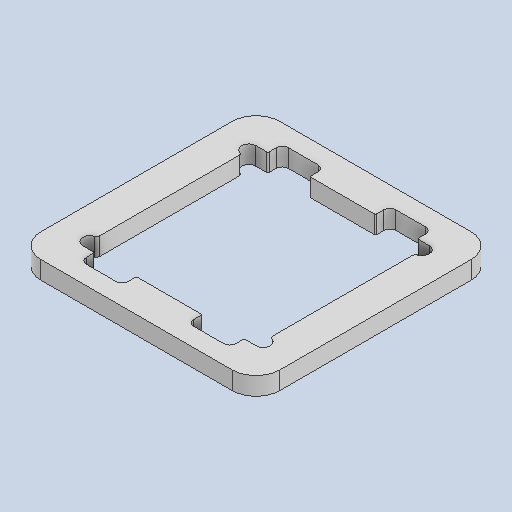
# Autodesk Inventor part: test switch hole
Saved by Autodesk Inventor 2025.2 (Build 292293000, 293)
## iProperties
Created: 2024-03-08
Part Number: test switch hole
Material: Generic
Document SubType Name: Modeling
Designer: mirun
Density: 1 g/cm^3
Appearance: Default
Author: mirun
Autodesk Inventor part; units mm, degrees
ref_plane "YZ Plane" through (0, 0, 0) normal (1, 0, 0) x (0, 1, 0)
ref_plane "XZ Plane" through (0, 0, 0) normal (0, 1, 0) x (-1, 0, 0)
ref_plane "XY Plane" through (0, 0, 0) normal (0, 0, 1) x (1, 0, 0)
sketch "Sketch1" plane through (0, 0, 0) normal (0, 1, 0) x (-1, 0, 0)
  line L0 (7.25, 5.8376) -> (7.25, -5.8376)
  line L1 (-7.25, -5.8376) -> (-7.25, 5.8376)
  line L2 (-7.25, 7.25) -> (7.25, -7.25) construction
  line L3 (7.25, 7.25) -> (-7.25, -7.25) construction
  line L4 (6.25, 7.25) -> (2.75, 7.25) construction
  line L5 (2.75, 7.35) -> (2.75, 7.95)
  line L6 (3.25, 8.45) -> (5.75, 8.45)
  line L7 (6.25, 7.95) -> (6.25, 7.35)
  arc A0 (7.4265, 6.0765) -> (7.25, 7.25) centre (7.25, 6.65) ccw
  line L8 (-7.25, 7.25) -> (2.65, 7.25)
  line L9 (6.35, 7.25) -> (7.25, 7.25)
  arc A1 (6.25, 7.35) -> (6.35, 7.25) centre (6.35, 7.35) ccw
  arc A2 (2.65, 7.25) -> (2.75, 7.35) centre (2.65, 7.35) ccw
  arc A3 (6.25, 7.95) -> (5.75, 8.45) centre (5.75, 7.95) ccw
  arc A4 (3.25, 8.45) -> (2.75, 7.95) centre (3.25, 7.95) ccw
  arc A5 (7.4265, 6.0765) -> (7.25, 5.8376) centre (7.5, 5.8376) ccw
  line L10 (0, 0) -> (2.8942, 0)
  line L11 (0, 0) -> (0, -4.9214)
  line L12 (7.25, -7.25) -> (-7.25, 7.25) construction
  line L13 (6.25, -7.25) -> (2.75, -7.25) construction
  line L14 (2.75, -7.35) -> (2.75, -7.95)
  line L15 (3.25, -8.45) -> (5.75, -8.45)
  line L16 (6.25, -7.95) -> (6.25, -7.35)
  arc A6 (7.25, -7.25) -> (7.4265, -6.0765) centre (7.25, -6.65) ccw
  line L17 (6.35, -7.25) -> (7.25, -7.25)
  arc A7 (6.35, -7.25) -> (6.25, -7.35) centre (6.35, -7.35) ccw
  arc A8 (2.75, -7.35) -> (2.65, -7.25) centre (2.65, -7.35) ccw
  arc A9 (5.75, -8.45) -> (6.25, -7.95) centre (5.75, -7.95) ccw
  arc A10 (2.75, -7.95) -> (3.25, -8.45) centre (3.25, -7.95) ccw
  arc A11 (7.25, -5.8376) -> (7.4265, -6.0765) centre (7.5, -5.8376) ccw
  line L18 (7.25, -7.25) -> (6.35, -7.25)
  line L19 (-6.25, 7.25) -> (-2.75, 7.25) construction
  line L20 (-2.75, 7.35) -> (-2.75, 7.95)
  line L21 (-3.25, 8.45) -> (-5.75, 8.45)
  line L22 (-6.25, 7.95) -> (-6.25, 7.35)
  arc A12 (-7.25, 7.25) -> (-7.4265, 6.0765) centre (-7.25, 6.65) ccw
  line L23 (-6.35, 7.25) -> (-7.25, 7.25)
  arc A13 (-6.35, 7.25) -> (-6.25, 7.35) centre (-6.35, 7.35) ccw
  arc A14 (-2.75, 7.35) -> (-2.65, 7.25) centre (-2.65, 7.35) ccw
  arc A15 (-5.75, 8.45) -> (-6.25, 7.95) centre (-5.75, 7.95) ccw
  arc A16 (-2.75, 7.95) -> (-3.25, 8.45) centre (-3.25, 7.95) ccw
  arc A17 (-7.25, 5.8376) -> (-7.4265, 6.0765) centre (-7.5, 5.8376) ccw
  arc A18 (-7.4265, -6.0765) -> (-7.25, -5.8376) centre (-7.5, -5.8376) ccw
  arc A19 (-7.4265, -6.0765) -> (-7.25, -7.25) centre (-7.25, -6.65) ccw
  line L24 (-6.35, -7.25) -> (-7.25, -7.25)
  line L25 (-7.25, -7.25) -> (7.25, 7.25) construction
  arc A20 (-6.25, -7.35) -> (-6.35, -7.25) centre (-6.35, -7.35) ccw
  line L26 (-6.25, -7.95) -> (-6.25, -7.35)
  arc A21 (-6.25, -7.95) -> (-5.75, -8.45) centre (-5.75, -7.95) ccw
  line L27 (-6.25, -7.25) -> (-2.75, -7.25) construction
  line L28 (-3.25, -8.45) -> (-5.75, -8.45)
  arc A22 (-2.65, -7.25) -> (-2.75, -7.35) centre (-2.65, -7.35) ccw
  line L29 (-2.75, -7.35) -> (-2.75, -7.95)
  arc A23 (-3.25, -8.45) -> (-2.75, -7.95) centre (-3.25, -7.95) ccw
  line L30 (-7.25, -7.25) -> (-6.35, -7.25)
  line L31 (2.65, -7.25) -> (-2.65, -7.25)
  line L32 (-6.35, -7.25) -> (-7.25, -7.25)
  line L33 (8, -10) -> (-8, -10)
  line L34 (-10, -8) -> (-10, 8)
  line L35 (-8, 10) -> (8, 10)
  line L36 (10, 8) -> (10, -8)
  arc A24 (10, 8) -> (8, 10) centre (8, 8) ccw
  arc A25 (8, -10) -> (10, -8) centre (8, -8) ccw
  arc A26 (-10, -8) -> (-8, -10) centre (-8, -8) ccw
  arc A27 (-8, 10) -> (-10, 8) centre (-8, 8) ccw
  point P0 (2.75, 8.45)
  point P1 (6.25, 8.45)
  point P2 (6.25, 7.65)
  point P3 (7.25, 6.05)
  point P4 (2.75, -8.45)
  point P5 (6.25, -8.45)
  point P6 (6.25, -7.65)
  point P7 (7.25, -6.05)
  point P8 (-2.75, 8.45)
  point P9 (-6.25, 8.45)
  point P10 (-6.25, 7.65)
  point P11 (-7.25, 6.05)
  point P12 (-7.25, -6.05)
  point P13 (-6.25, -7.65)
  point P14 (-6.25, -8.45)
  point P15 (-2.75, -8.45)
  point P16 (10, -10)
  point P17 (-10, -10)
  point P18 (-10, 10)
  point P19 (10, 10)
  point P20 (-7.25, 7.25)
  point P21 (-6.35, 7.25)
  point P22 (-2.65, 7.25)
  dimension "d0" = 14.5
  dimension "d1" = 14.5
  dimension "d2" = 3.5
  dimension "d3" = 1.2
  dimension "d4" = 1
  dimension "d5" = 1.2
  dimension "d6" = 0.1
  dimension "d7" = 0.1
  dimension "d8" = 0.5
  dimension "d9" = 0.25
  dimension "d10" = 2
  dimension "d13" = 20
  dimension "d14" = 20
  constraints: 74 end point, 68 symmetric about line, 60 point on circle, 39 point on line, 28 centre point, 20 tangent, 9 parallel, 5 midpoint, 4 equal radius, 4 horizontal, 4 perpendicular, 27 other
  measures "d0" distance of L2.end L3.end
  measures "d1" distance of L3.start L2.end
  measures "d2" distance of point (2.75, 8.45) point (6.25, 8.45)
  measures "d3" distance of L4.end point (2.75, 8.45)
  measures "d4" distance from line of L0 point (6.25, 7.65)
  measures "d5" diameter of A0
  measures "d6" radius of A1
  measures "d7" radius of A2
  measures "d8" radius of A3
  measures "d9" radius of A5
  measures "d10" radius of A24
  measures "d13" distance between parallel lines of L34 L36
  measures "d14" distance between parallel lines of L35 L33
extrude "Extrusion1" add sketch "Sketch1" along normal blind 1.5
body "Solid1"
